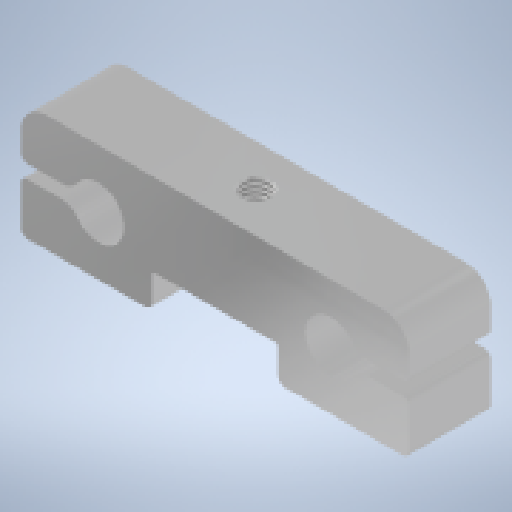
# Autodesk Inventor part: Printhead Belt Retainer
Saved by Autodesk Inventor 2024 (Build 280153000, 153)
## iProperties
Created: 2024-12-29
Part Number: Printhead Belt Retainer
Material: Aluminum 6061
Document SubType Name: Modeling
Designer: Ishaan
Density: 2.7 g/cm^3
Appearance: Aluminum - Flat
Author: Ishaan
Autodesk Inventor part; units mm, degrees
ref_plane "YZ Plane" through (0, 0, 0) normal (1, 0, 0) x (0, 1, 0)
ref_plane "XZ Plane" through (0, 0, 0) normal (0, 1, 0) x (-1, 0, 0)
ref_plane "XY Plane" through (0, 0, 0) normal (0, 0, 1) x (1, 0, 0)
sketch "Sketch1" plane through (0, 0, 0) normal (0, 0, 1) x (1, 0, 0)
  line L0 (30, -9) -> (-30, -9)
  line L1 (-30, -9) -> (-30, 9)
  line L2 (-30, 9) -> (30, 9)
  line L3 (30, 9) -> (30, -9)
  line L4 (30, -9) -> (-30, 9) construction
  line L5 (-30, -9) -> (30, 9) construction
  circle A0 centre (-18, 0) radius 4
  circle A1 centre (18, 0) radius 4
  line L6 (-18, 0) -> (18, 0) construction
  line L7 (30, -1.05) -> (-30, -1.05)
  line L8 (-30, -1.05) -> (-30, 1.05) construction
  line L9 (-30, 1.05) -> (30, 1.05)
  line L10 (30, 1.05) -> (30, -1.05) construction
  line L11 (30, -1.05) -> (-30, 1.05) construction
  line L12 (-30, -1.05) -> (30, 1.05) construction
  point P0 (0, 0)
  point P1 (-21.8597, 1.05)
  point P2 (-21.8597, -1.05)
  point P3 (21.8597, -1.05)
  point P4 (21.8597, 1.05)
  dimension "d0" = 60
  dimension "d1" = 18
  dimension "d2" = 8
  dimension "d4" = 2.1
  dimension "d5" = 36
  constraints: 26 end point, 5 midpoint, 4 parallel, 3 horizontal, 2 centre point, 2 perpendicular, 1 equal radius, 1 point on line
  measures "d0" distance of L1.end L2.end
  measures "d1" distance of L0.end L1.end
  measures "d2" diameter of A0
  measures "d4" distance of L7.end L8.end
  measures "d5" distance of L6.start L6.end
extrude "Extrusion1" add sketch "Sketch1" along normal blind 12.7 contours L0 L1 L7 A0 A1 L3 | L9 A1 A0 L1 L2 L3 | L7 A0 L9 A1
fillet "Fillet1" radius 3 4 edges at (-21.8597, 1.05, 6.35) (-21.8597, -1.05, 6.35) (21.8597, 1.05, 6.35) (21.8597, -1.05, 6.35)
sketch "Sketch2" plane through (0, 0, 12.7) normal (0, 0, 1) x (1, 0, 0)
  line L0 (9.75, -9) -> (-9.75, -9)
  line L1 (-9.75, -9) -> (-9.75, -3.725)
  line L2 (-9.75, -3.725) -> (9.75, -3.725)
  line L3 (9.75, -3.725) -> (9.75, -9)
  line L4 (9.75, -9) -> (-9.75, -3.725) construction
  line L5 (-9.75, -9) -> (9.75, -3.725) construction
  line L6 (-30, -9) -> (30, -9) projected
  arc A0 (-21.2625, -2.3143) -> (-21.2625, 2.3143) centre (-18, 0) ccw projected
  circle A1 centre (-18, 0) radius 9.052 construction
  point P0 (0, 0)
  point P1 (0, -6.3625)
  dimension "d9" = 3.725
  dimension "d10" = 5.052
  dimension "d11" = 19.5
  constraints: 12 end point, 2 midpoint, 2 parallel, 1 coincident, 1 collinear, 1 horizontal, 1 perpendicular, 1 vertical alignment, 3 other
  measures "d9" distance from line of point (0, 0) L2
  measures "d11" distance of L1.end L2.end
extrude "Extrusion2" cut sketch "Sketch2" against normal up to surface (12.7 mm away)
fillet "Fillet2" radius 1 4 edges at (9.75, -9, 6.35) (-9.75, -9, 6.35) (-30, -9, 6.35) (30, -9, 6.35)
fillet "Fillet3" radius 4 2 edges at (30, 9, 6.35) (-30, 9, 6.35)
fillet "Fillet4" radius 1 4 edges at (-30, 1.05, 6.35) (-30, -1.05, 6.35) (30, 1.05, 6.35) (30, -1.05, 6.35)
fillet "Fillet5" radius 0.5 2 edges at (9.75, -3.725, 6.35) (-9.75, -3.725, 6.35)
sketch "Sketch3" plane through (-9.25, -3.725, 12.7) normal (0, -1, 0) x (1, 0, 0)
  line L0 (0, -12.7) -> (0, 0) projected
  line L1 (18.5, -12.7) -> (0, -12.7) projected
  line L2 (18.5, 0) -> (18.5, -12.7) projected
  line L3 (0, 0) -> (18.5, 0) projected
  line L4 (9.25, -12.7) -> (9.25, 0) construction
  point P0 (9.25, -6.35)
  constraints: 2 end point, 2 midpoint
hole "Hole1" at (0, -3.725, 6.35) direction (0, 1, 0) diameter 4.134 end through all thread size "M5x0.8" class "6H" standard "ANSI Metric M Profile"
chamfer "Chamfer1" distance 0.25 angle 45 2 edges at (0, 9, 8.417) (0, -3.725, 8.417)
body "Solid1"
